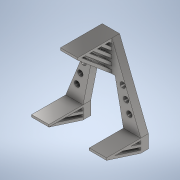
# Autodesk Inventor part: Soporte
Saved by Autodesk Inventor 2021 (Build 250183000, 183)
## iProperties
Created: 2021-07-01
Part Number: Soporte
Material: Acero inoxidable 302 AISI
Document SubType Name: Modeling
Designer: Alma
Density: 8 g/cm^3
Appearance: Semipulido
Mass: 23040.5 g
Surface Area: 3926.97 cm^2
Volume: 2880.06 cm^3
Author: Alma
Autodesk Inventor part; units mm, degrees
ref_plane "YZ Plane" through (0, 0, 0) normal (1, 0, 0) x (0, 1, 0)
ref_plane "XZ Plane" through (0, 0, 0) normal (0, 1, 0) x (-1, 0, 0)
sketch "Boceto7" plane through (0, 0, 0) normal (0, 0, 1) x (1, 0, 0)
  line L0 (0, 0) -> (342, 0)
  line L1 (171, 330.115) -> (171, 0) construction
  line L2 (131.5, 347.5309) -> (210.5, 347.5309) construction
  line L3 (210.5, 330.115) -> (131.5, 330.115)
  line L4 (0, 0) -> (131.5, 330.115)
  line L5 (342, 0) -> (210.5, 330.115)
  line L6 (0, 0) -> (0, -10) construction
  line L7 (0, -10) -> (78.602, -10) construction
  line L8 (0, -10) -> (78.602, -10)
  line L9 (0, -10) -> (0, 0)
  line L10 (78.602, -10) -> (342, -10)
  line L11 (342, -10) -> (342, 0)
  line L12 (131.5, 330.115) -> (131.5, 320.115)
  line L13 (131.5, 320.115) -> (210.5, 320.115)
  line L14 (210.5, 320.115) -> (210.5, 330.115)
  line L15 (78.602, -10) -> (78.602, 0)
  line L16 (263.398, -10) -> (263.398, 0)
  line L17 (0, -10) -> (78.602, -10)
  line L18 (78.602, -10) -> (78.602, -60)
  line L19 (78.602, -60) -> (0, -60)
  line L20 (0, -60) -> (0, -10)
  line L21 (263.398, -10) -> (263.398, -60)
  line L22 (263.398, -60) -> (342, -60)
  line L23 (342, -60) -> (342, -10)
  line L24 (78.602, 0) -> (116.5722, 189.115)
  line L25 (116.5722, 189.115) -> (225.4278, 189.115)
  line L26 (225.4278, 189.115) -> (263.398, 0)
  point P0 (263.398, 0)
  point P1 (263.398, -10)
  dimension "d68" = 79
  dimension "d69" = 39.5
  dimension "d70" = 342
  dimension "d71" = 330.115
  dimension "d72" = 10
  dimension "d73" = 78.602
  dimension "d74" = 10
  dimension "d111" = 50
  dimension "d144" = 141
  constraints: 54 end point, 7 perpendicular, 6 horizontal, 5 symmetric about line, 3 parallel, 1 collinear, 1 midpoint, 1 point on line, 1 vertical
  measures "d68" distance of L2.start L2.end
  measures "d69" horizontal distance of L1.start L2.start
  measures "d70" distance of L0.start L0.end
  measures "d71" distance of L1.start L1.end
  measures "d72" distance of L0.start L6.end
  measures "d73" distance of L6.end L7.end
  measures "d74" distance of L3.end L12.end
  measures "d111" distance of L17.end L18.end
  measures "d144" distance between parallel lines of L3 L25
extrude "Extrusión5" add sketch "Boceto7" along normal blind 35 contours L4 L12 L13 L14 L5 L0 L26 L25 L24 | L0 L15 L8 L9 | L3 L14 L13 L12 | L8 L18 L19 L20 | L0 L11 L10 L16 | L10 L23 L22 L21
extrude "Extrusión6" add sketch "Boceto7" along normal blind 191 contours L0 L15 L8 L9 | L3 L14 L13 L12 | L0 L11 L10 L16
ref_plane "Plano de trabajo2" through (171, -60, 0) normal (1, 0, 0) x (0, 0, -1)
sketch "Boceto12" plane through (171, -60, 0) normal (1, 0, 0) x (0, 0, -1)
  line L0 (-35, 380.115) -> (-191, 380.115) projected
  line L1 (-191, 380.115) -> (-35, 249.2155)
  line L2 (-35, 390.115) -> (-35, 60) projected
  line L3 (-173.0135, 380.115) -> (-35, 264.3079)
  line L4 (-173.0135, 395.115) -> (-35, 279.3079)
  line L5 (-173.0135, 410.115) -> (-35, 294.3079)
  line L6 (-173.0135, 425.115) -> (-35, 309.3079)
  line L7 (-173.0135, 440.115) -> (-35, 324.3079)
  line L8 (-173.0135, 455.115) -> (-35, 339.3079)
  line L9 (-173.0135, 470.115) -> (-35, 354.3079)
  line L10 (-173.0135, 485.115) -> (-35, 369.3079)
  line L11 (-173.0135, 500.115) -> (-35, 384.3079)
  line L12 (-173.0135, 515.115) -> (-35, 399.3079)
  line L13 (-173.0135, 530.115) -> (-35, 414.3079)
  line L14 (-35, 60) -> (-35, 390.115) projected
  line L15 (138.0135, 380.115) -> (138.0135, 210.115) construction
  point P0 (0, 60)
  point P1 (-10, 338.3304)
  point P2 (-23.0135, 325.115)
  point P3 (-12.1268, 325.115)
  point P4 (-30, 350.1124)
  point P5 (-30.0031, 385.115)
  point P6 (-47.8794, 380.115)
  point P7 (-65.7557, 380.115)
  point P8 (-83.632, 380.115)
  point P9 (-101.5083, 380.115)
  point P10 (-119.3846, 380.115)
  point P11 (-137.2609, 380.115)
  point P12 (-155.1372, 380.115)
  dimension "d90" = 40
  dimension "d93" = 15
  dimension "d107" = 170
  dimension "d108" = 0
  constraints: 26 end point, 3 point on line, 2 vertical, 1 parallel, 31 other
  measures "d90" angle of L0 L1
  measures "d93" distance of L3.start L4.start
  measures "d107" distance of L15.start L15.end
  measures "d108" distance from line of L15.start L0
extrude "Extrusión9" add sketch "Boceto12" along normal mid plane 79 contours L3 L2 L1 L0 | L0 L5 L2 L4 | L0 L7 L2 L6 | L0 L9 L2 L8 | L0 L2 L10
sketch "Boceto13" plane through (0, 0, 35) normal (0, 0, 1) x (1, 0, 0)
  circle A0 centre (81.5, 169.115) radius 12.7
  circle A1 centre (66.5, 119.115) radius 12.7
  circle A2 centre (51.5, 69.115) radius 12.7
  line L0 (116.5722, 189.115) -> (225.4278, 189.115) projected
  line L1 (131.5, 189.2155) -> (131.5, 320.115) projected
  line L2 (131.5, 320.115) -> (210.5, 320.115) construction
  line L3 (171, 320.115) -> (171, 34.3684) construction
  circle A3 centre (260.5, 169.115) radius 12.7
  circle A4 centre (275.5, 119.115) radius 12.7
  circle A5 centre (290.5, 69.115) radius 12.7
  point P0 (131.5, 193.411)
  dimension "d126" = 25.4
  dimension "d127" = 25.4
  dimension "d128" = 25.4
  dimension "d129" = 20
  dimension "d130" = 50
  dimension "d131" = 50
  dimension "d132" = 50
  dimension "d133" = 65
  dimension "d134" = 80
  constraints: 6 centre point, 3 symmetric about line, 2 end point, 1 midpoint, 1 vertical, 3 other
  measures "d126" diameter of A0
  measures "d127" diameter of A1
  measures "d128" diameter of A2
  measures "d129" distance from line of A0.centre L0
  measures "d130" vertical distance of A0.centre A1.centre
  measures "d131" vertical distance of A1.centre A2.centre
  measures "d132" distance from line of L1 A0.centre
  measures "d133" distance from line of L1 A1.centre
  measures "d134" distance from line of L1 A2.centre
extrude "Extrusión10" cut sketch "Boceto13" against normal up to surface (35 mm away)
sketch "Boceto16" plane through (342, -60, 0) normal (1, 0, 0) x (0, 0, -1)
  line L0 (-191, 50) -> (-191, 60) projected
  line L1 (0, 0) -> (-35, 0) projected
  line L2 (-191, 50) -> (-35, 0)
  line L3 (-35, 0) -> (-35, 50) projected
  line L4 (-191, 62) -> (-35, 12)
  line L5 (-191, 74) -> (-35, 24)
  line L6 (-191, 86) -> (-35, 36)
  line L7 (-191, 98) -> (-35, 48)
  line L8 (-191, 110) -> (-35, 60)
  line L9 (-35, 50) -> (-191, 50) projected
  point P0 (0, 60)
  point P1 (-78.68, 50)
  point P2 (-116.12, 50)
  point P3 (-153.56, 50)
  dimension "d137" = 12
  constraints: 12 end point, 1 vertical, 15 other
  measures "d137" distance of L0.start L4.start
extrude "Extrusión13" add sketch "Boceto16" against normal blind 79 contours L9 L4 L3 L2 | L9 L6 L3 L5
mirror "Simetría2" about plane through (171, -60, 0) normal (1, 0, 0) of "Extrusión13"
thread "Rosca1" size "M26x1.5" class "6H" standard "ANSI Metric M Profile" full length
thread "Rosca2" size "M26x1.5" class "6H" standard "ANSI Metric M Profile" full length
thread "Rosca3" size "M26x1.5" class "6H" standard "ANSI Metric M Profile" full length
thread "Rosca4" size "M26x1.5" class "6H" standard "ANSI Metric M Profile" full length
thread "Rosca5" size "M26x1.5" class "6H" standard "ANSI Metric M Profile" full length
thread "Rosca6" size "M26x1.5" class "6H" standard "ANSI Metric M Profile" full length
